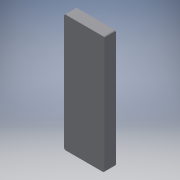
# Autodesk Inventor part: Supporter
Saved by Autodesk Inventor 2018 (Build 220112000, 112)
## iProperties
Created: 2017-12-13
Part Number: Supporter
Material: Generic
Document SubType Name: Modeling
Designer: kcmat
Density: 1 g/cm^3
Appearance: Default
Author: kcmat
Autodesk Inventor part; units mm, degrees
ref_plane "YZ Plane" through (0, 0, 0) normal (1, 0, 0) x (0, 1, 0)
ref_plane "XZ Plane" through (0, 0, 0) normal (0, 1, 0) x (-1, 0, 0)
sketch "Sketch1" plane through (0, 0, 0) normal (0, 0, 1) x (1, 0, 0)
  line L0 (165.7182, 252.0837) -> (146.6642, 252.0837) projected
  line L1 (158.6327, 216.5237) -> (165.7182, 216.5237) projected
  line L2 (139.5562, 216.5237) -> (143.6242, 216.5237) projected
  line L3 (143.6242, 252.0837) -> (139.5562, 252.0837) projected
  line L4 (126.4117, 267.0247) -> (136.1907, 267.0247) projected
  line L5 (136.1907, 190.8247) -> (126.4117, 190.8247) projected
  line L6 (139.5562, 267.0247) -> (139.5562, 190.8247)
  line L7 (139.5562, 190.8247) -> (165.7182, 190.8247)
  line L8 (165.7182, 190.8247) -> (165.7182, 267.0247)
  line L9 (165.7182, 267.0247) -> (139.5562, 267.0247)
  point P0 (0, 0)
  constraints: 8 end point, 3 perpendicular, 1 vertical
ref_plane "Work Plane1" through (146.6642, 216.5237, 7.3936) normal (0, 0, -1) x (0, 1, 0)
extrude "Extrusion1" add sketch "Sketch1" along normal up to surface (7.3936 mm away)
fillet "Fillet1" radius 1 4 edges at (139.5562, 190.8247, 3.6968) (139.5562, 267.0247, 3.6968) (165.7182, 267.0247, 3.6968) (165.7182, 190.8247, 3.6968)
sketch "Sketch3" plane through (0, 0, 0) normal (0, 0, -1) x (-1, 0, 0)
  circle A0 centre (-160.3842, 185.8247) radius 1.25
  line L0 (-165.7182, 191.8247) -> (-165.7182, 194.8247)
  line L1 (-165.7182, 191.8247) -> (-165.7182, 266.0247) projected
  line L2 (-165.7182, 194.8247) -> (-161.7182, 194.8247)
  circle A1 centre (-161.7182, 194.8247) radius 1.25
  line L3 (-140.5562, 190.8247) -> (-164.7182, 190.8247) projected
  line L4 (-165.7182, 228.9247) -> (-156.0588, 228.9247)
  line L5 (-152.6372, 190.8247) -> (-152.6372, 206.7203)
  line L6 (-139.5562, 191.8247) -> (-139.5562, 194.8247)
  line L7 (-139.5562, 191.8247) -> (-139.5562, 266.0247)
  line L8 (-139.5562, 194.8247) -> (-143.5562, 194.8247)
  circle A2 centre (-143.5562, 194.8247) radius 1.25
  line L9 (-164.7182, 190.8247) -> (-140.5562, 190.8247)
  circle A3 centre (-160.3842, 272.0247) radius 1.25
  line L10 (-165.7182, 266.0247) -> (-165.7182, 263.0247)
  line L11 (-165.7182, 266.0247) -> (-165.7182, 191.8247)
  line L12 (-165.7182, 263.0247) -> (-161.7182, 263.0247)
  circle A4 centre (-161.7182, 263.0247) radius 1.25
  line L13 (-140.5562, 267.0247) -> (-164.7182, 267.0247)
  line L14 (-152.6372, 267.0247) -> (-152.6372, 251.1291)
  line L15 (-139.5562, 266.0247) -> (-139.5562, 263.0247)
  line L16 (-139.5562, 266.0247) -> (-139.5562, 191.8247)
  line L17 (-139.5562, 263.0247) -> (-143.5562, 263.0247)
  circle A5 centre (-143.5562, 263.0247) radius 1.25
  line L18 (-164.7182, 267.0247) -> (-140.5562, 267.0247)
  point P0 (0, 0)
  dimension "d11" = 3
  dimension "d12" = 4
  dimension "d13" = 2.5
  dimension "d14" = 4
  constraints: 34 end point, 27 symmetric about line, 6 centre point, 4 coincident, 4 point on line, 2 horizontal, 2 midpoint, 1 vertical, 6 other
  measures "d11" distance of L0.start L0.end
  measures "d12" distance of L0.end L2.end
  measures "d13" diameter of A1
  measures "d14" distance between parallel lines of L2 L3
extrude "Extrusion3" cut sketch "Sketch3" against normal blind 5 contours A4 | A1 | A5 | A2
body "Solid1"
